stdeqnema17 (Autodesk Fusion 360 design; units mm, degrees)
Autodesk Fusion 360 part; units mm, degrees
sketch "Esquisse1" plane through (0, 0, 0) normal (0, 0, 1) x (1, 0, 0)
  line L0 (0, 0) -> (50, 0)
  line L1 (50, 0) -> (50, 50)
  line L2 (50, 50) -> (0, 50)
  line L3 (0, 50) -> (0, 0)
  dimension "d1" = 50
  dimension "d2" = 50
  constraint horizontal L0
  constraint vertical L1
  constraint horizontal L2
  constraint vertical L3
  constraint coincident L0.start L3.end
  measures "d1" distance of L1.end L2.end
  measures "d2" distance of L0.end L1.end
extrude "Extrusion1" add sketch "Esquisse1" along normal blind 2.7
sketch "Esquisse2" plane through (0, 0, 0) normal (0, 1, 0) x (1, 0, 0)
  line L0 (0, -50) -> (50, -50)
  line L1 (50, -50) -> (50, 0)
  line L2 (50, 0) -> (0, 0)
  line L3 (0, 0) -> (0, -50)
  constraint horizontal L0
  constraint vertical L1
  constraint horizontal L2
  constraint vertical L3
extrude "Extrusion2" add sketch "Esquisse2" against normal blind 2.7
sketch "Esquisse3" plane through (0, 0, 2.7) normal (0, 0, 1) x (-1, 0, 0)
  line L0 (0, -50) -> (0, 0)
  line L1 (0, 0) -> (-50, 0)
  line L2 (-50, 0) -> (-50, -50)
  line L3 (-50, -50) -> (0, -50)
  circle A0 centre (-25, -25) radius 11
  dimension "d7" = 22
  measures "d7" diameter of A0
extrude "Extrusion3" cut sketch "Esquisse3" against normal blind 10 contours A0
sketch "Esquisse4" plane through (0, 0, 2.7) normal (0, 0, 1) x (-1, 0, 0)
  circle A0 centre (-25, -25) radius 11
  line L0 (0, -50) -> (0, 0)
  line L1 (0, 0) -> (-50, 0)
  line L2 (-50, 0) -> (-50, -50)
  line L3 (-50, -50) -> (0, -50)
  circle A1 centre (-9.5, -40.5) radius 2
  dimension "d10" = 4
  dimension "d11" = 15.5
  dimension "d12" = 15.5
  measures "d10" diameter of A1
  measures "d11" vertical distance of A0.centre A1.centre
  measures "d12" horizontal distance of A0.centre A1.centre
extrude "Extrusion4" cut sketch "Esquisse4" against normal blind 10 contours A1
pattern_linear "Réseau R1" count 2 spacing 31 along (1, 0, 0) count 2 spacing 31 along (0, -1, 0) of "Extrusion4"
sketch "Esquisse5" plane through (0, 0, 0) normal (0, 1, 0) x (-1, 0, 0)
  line L0 (-50, 2.7) -> (0, 2.7)
  line L1 (0, 2.7) -> (0, 50)
  line L2 (0, 50) -> (-50, 50)
  line L3 (-50, 50) -> (-50, 2.7)
  line L4 (-42.65, 9.1521) -> (-42.65, 43.1521)
  arc A0 (-38.35, 43.1521) -> (-42.65, 43.1521) centre (-40.5, 43.1521) ccw
  line L5 (-38.35, 43.1521) -> (-38.35, 9.1521)
  arc A1 (-42.65, 9.1521) -> (-38.35, 9.1521) centre (-40.5, 9.1521) ccw
  dimension "d19" = 4.3
  dimension "d20" = 34
  dimension "d22" = 9.5
  constraint vertical L4
  constraint tangent L4 A0
  constraint parallel L4 L5
  constraint tangent L4 A1
  constraint tangent L5 A1
  constraint tangent A0 L5
  measures "d19" distance of L4 L5
  measures "d20" distance of L4.start L4.end
  measures "d22" distance of L3 A0.centre
extrude "Extrusion5" cut sketch "Esquisse5" against normal blind 6 contours L4 A0 L5 A1
pattern_linear "Réseau R2" count 2 spacing 31 along (-1, 0, 0) of "Extrusion5"
chamfer "Chanfrein1" distance 4 angle 45 4 edges at (50, -1.35, 50) (0, -1.35, 50) (50, 50, 1.35) (0, 50, 1.35)
equation "d11 = ( 31 / 2 ) * 1 mm"
equation "d12 = ( 31 / 2 ) * 1 mm"
